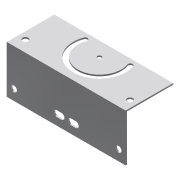
# Autodesk Inventor part: L profil
Saved by Autodesk Inventor 2015 (Build 190159000, 159)
## iProperties
Created: 2015-01-07
Part Number: L profil
Material: Všeobecné
Document SubType Name: Modeling
Designer: Michal
Density: 1 g/cm^3
Appearance: Hliník – leštěný
Author: Michal
Autodesk Inventor part; units mm, degrees
ref_plane "YZ Plane" through (0, 0, 0) normal (1, 0, 0) x (0, 1, 0)
ref_plane "XZ Plane" through (0, 0, 0) normal (0, 1, 0) x (-1, 0, 0)
ref_plane "XY Plane" through (0, 0, 0) normal (0, 0, 1) x (1, 0, 0)
sketch "Náčrt1" plane through (0, 0, 0) normal (1, 0, 0) x (0, 1, 0)
  line L0 (0, 0) -> (100, 0)
  line L1 (100, 0) -> (100, -3)
  line L2 (100, -3) -> (3, -3)
  line L3 (3, -3) -> (3, -100)
  line L4 (3, -100) -> (0, -100)
  line L5 (0, -100) -> (0, 0)
  point P0 (100, -148)
  point P1 (100, -150)
  dimension "d0" = 100
  dimension "d1" = 3
  dimension "d20" = 100
  dimension "d40" = 3
  dimension "d41" = 97
  dimension "d42" = 97
  constraints: 12 end point, 3 perpendicular, 2 point on line, 1 horizontal
  measures "d0" distance of L0.start L0.end
  measures "d1" distance of L0.end L1.end
  measures "d20" distance of L4.end L0.start
  measures "d40" distance of L3.end L4.end
  measures "d41" distance of L2.end L3.end
  measures "d42" distance of L1.end L2.end
extrude "Vysunutí1" add sketch "Náčrt1" along normal blind 140
sketch "Náčrt7" plane through (0, 3, -3) normal (0, 0, -1) x (-1, 0, 0)
  circle A0 centre (-125, 21) radius 6.25
  line L0 (0, 0) -> (-140, 0) projected
  line L1 (-140, 0) -> (-140, 97) projected
  line L2 (0, 97) -> (0, 0) projected
  point P0 (0, -3)
  dimension "d43" = 12.5
  dimension "d44" = 21
  dimension "d101" = 15
  constraints: 1 centre point
  measures "d43" diameter of A0
  measures "d44" distance from line of A0.centre L0
  measures "d101" distance from line of L1 A0.centre
extrude "Vysunutí6" cut sketch "Náčrt7" against normal through all
sketch "Náčrt11" plane through (0, 0, 0) normal (-1, 0, 0) x (0, 0, 1)
  line L0 (0, 0) -> (0, 100) projected
  line L1 (0, 100) -> (-3, 100) projected
  line L2 (-3, 100) -> (-3, 3) projected
  line L3 (-3, 3) -> (-100, 3) projected
  line L4 (-100, 3) -> (-100, 0) projected
  line L5 (-100, 0) -> (0, 0) projected
extrude "Vysunutí9" add sketch "Náčrt11" along normal blind 110
sketch "Náčrt9" plane through (0, 3, -3) normal (0, 1, 0) x (1, 0, 0)
  line L0 (140, 97) -> (-110, 97) projected
  line L1 (140, -3) -> (140, 97) projected
  line L2 (-110, -3) -> (140, -3) projected
  line L3 (0, -3) -> (140, -3) projected
  arc A0 (5, 68.75) -> (5, 81.25) centre (5, 75) ccw
  arc A1 (-5, 81.25) -> (-5, 68.75) centre (-5, 75) ccw
  line L4 (-5, 68.75) -> (5, 68.75)
  line L5 (5, 81.25) -> (-5, 81.25)
  line L6 (-110, 97) -> (-110, -3) projected
  point P0 (0, 75)
  dimension "d89" = 140
  dimension "d91" = 12.5
  dimension "d92" = 12.5
  dimension "d93" = 10
  dimension "d94" = 5
  constraints: 4 end point, 4 point on circle, 2 centre point, 1 parallel, 1 tangent
  measures "d89" distance from line of L1 point (0, 75)
  measures "d91" diameter of A0
  measures "d92" diameter of A1
  measures "d93" distance of A1.centre A0.centre
  measures "d94" distance of point (0, 75) A0.centre
sketch "Náčrt10" plane through (0, 0, 0) normal (0, 0, 1) x (1, 0, 0)
  line L0 (0, 100) -> (140, 100) projected
  circle A0 centre (125, 24) radius 6.25 projected
  circle A1 centre (15, 70) radius 4.25
  arc A2 (-27.756, 85.5619) -> (57.756, 85.5619) centre (15, 70) ccw
  arc A3 (-37.1529, 88.9821) -> (67.1529, 88.9821) centre (15, 70) ccw
  arc A4 (67.1529, 88.9821) -> (57.756, 85.5619) centre (62.4545, 87.272) ccw
  line L1 (15, 70) -> (84.9162, 70)
  line L2 (15, 70) -> (58.1675, 85.7117)
  line L3 (15, 70) -> (15, -7.5844)
  line L4 (15, 70) -> (-27.756, 85.5619)
  arc A5 (-27.756, 85.5619) -> (-37.1529, 88.9821) centre (-32.4545, 87.272) ccw
  line L5 (140, 100) -> (140, 0) projected
  line L6 (0, 0) -> (140, 0) projected
  dimension "d66" = 8.5
  dimension "d67" = 91
  dimension "d68" = 111
  dimension "d69" = 10
  dimension "d70" = 10
  dimension "d73" = 20
  dimension "d74" = 110
  dimension "d78" = 10
  dimension "d83" = 125
  dimension "d84" = 70
  constraints: 8 end point, 8 point on circle, 5 centre point, 2 coincident, 2 tangent, 1 horizontal, 1 point on line, 1 vertical
  measures "d66" diameter of A1
  measures "d67" diameter of A2
  measures "d68" diameter of A3
  measures "d69" radial gap between concentric circles of A3 A2
  measures "d70" diameter of A4
  measures "d73" angle of L1 L2
  measures "d74" angle of L3 L4
  measures "d78" diameter of A5
  measures "d83" distance from line of L5 A1.centre
  measures "d84" distance from line of L6 A1.centre
extrude "Vysunutí13" cut sketch "Náčrt9" against normal through all contours L4 A1 L5 A0
extrude "Vysunutí14" cut sketch "Náčrt10" against normal through all contours L1 L2 A1 | A1 L3 L1 | L2 L4 A1 | A1 L4 L3 | L1 A3 L3 A2 | A2 A4 A3 L1 | L3 A3 A5 A2
ref_plane "Pracovní rovina2" through (15, 0, 0) normal (1, 0, 0) x (0, 0, -1)
mirror "Zrcadlit2" about plane through (15, 0, 0) normal (1, 0, 0) of "Vysunutí13", "Vysunutí6"
sketch "Náčrt12" plane through (140, 3, -3) normal (0, 1, 0) x (1, 0, 0)
  line L0 (-115, 81.25) -> (-105, 81.25) projected
  arc A0 (-105, 68.75) -> (-105, 81.25) centre (-105, 75) ccw projected
  line L1 (-105, 68.75) -> (-115, 68.75) projected
  arc A1 (-115, 81.25) -> (-115, 68.75) centre (-115, 75) ccw projected
  line L2 (-135, 68.75) -> (-145, 68.75) projected
  arc A2 (-145, 81.25) -> (-145, 68.75) centre (-145, 75) ccw projected
  line L3 (-145, 81.25) -> (-135, 81.25) projected
  arc A3 (-135, 68.75) -> (-135, 81.25) centre (-135, 75) ccw projected
  line L4 (0, 0) -> (-250, 0) projected
  line L5 (0, 97) -> (0, 0) projected
  line L6 (0, 97) -> (-250, 97) projected
  line L7 (-250, 0) -> (-250, 97) projected
  circle A4 centre (-15, 75) radius 6.25
  point P0 (-140, -3)
  dimension "d102" = 12.5
  dimension "d103" = 15
  constraints: 1 centre point
  measures "d102" diameter of A4
  measures "d103" distance from line of L5 A4.centre
extrude "Vysunutí15" cut sketch "Náčrt12" against normal through all contours A4
mirror "Zrcadlit3" about plane through (15, 0, 0) normal (1, 0, 0) of "Vysunutí15"
